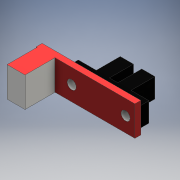
# Autodesk Inventor part: optical endstop
Saved by Autodesk Inventor 2016 SP1 (Build 200210100, 210)
## iProperties
Created: 2016-04-16
Part Number: optical endstop
Material: Generic
Document SubType Name: Modeling
Designer: ubik
Density: 1 g/cm^3
Appearance: Default
Author: ubik
Autodesk Inventor part; units mm, degrees
ref_plane "YZ Plane" through (0, 0, 0) normal (1, 0, 0) x (0, 1, 0)
ref_plane "XZ Plane" through (0, 0, 0) normal (0, 1, 0) x (-1, 0, 0)
ref_plane "XY Plane" through (0, 0, 0) normal (0, 0, 1) x (1, 0, 0)
sketch "Sketch1" plane through (0, 0, 0) normal (0, 0, 1) x (1, 0, 0)
  line L0 (-11.8, 0) -> (-11.8, 3)
  line L1 (-11.8, 3) -> (-5.8, 3)
  line L2 (-5.8, 3) -> (-5.8, 11)
  line L3 (-5.8, 11) -> (-1.4, 11)
  line L4 (-1.4, 11) -> (-1.4, 3)
  line L5 (-1.4, 3) -> (1.4, 3)
  line L6 (1.4, 3) -> (1.4, 11)
  line L7 (1.4, 11) -> (5.8, 11)
  line L8 (5.8, 11) -> (5.8, 3)
  line L9 (5.8, 3) -> (11.8, 3)
  line L10 (11.8, 3) -> (11.8, 0)
  line L11 (11.8, 0) -> (-11.8, 0)
  point P0 (0, 0)
  dimension "d0" = 3
  dimension "d1" = 6
  dimension "d2" = 8
  dimension "d3" = 4.4
  dimension "d4" = 2.8
  dimension "d5" = 4.4
  dimension "d6" = 6
  dimension "d7" = 1.4
  dimension "d8" = 0
  constraints: 24 end point, 8 perpendicular, 6 point on line, 1 vertical
  measures "d0" distance of L0.start L0.end
  measures "d1" distance of L0.end L1.end
  measures "d2" distance of L1.end L2.end
  measures "d3" distance of L2.end L3.end
  measures "d4" distance of L4.end L5.end
  measures "d5" distance of L6.end L7.end
  measures "d6" distance of L8.end L9.end
  measures "d7" distance from line of point (0, 0) L4
  measures "d8" distance from line of point (0, 0) L11
extrude "Extrusion1" add sketch "Sketch1" along normal blind 6.5
sketch "Sketch2" plane through (-11.8, 0, 0) normal (0, -1, 0) x (1, 0, 0)
  circle A0 centre (2.8, 3.25) radius 1.5
  circle A1 centre (20.8, 3.25) radius 1.5
  line L0 (23.6, 0) -> (23.6, 6.5) projected
  line L1 (0, 0) -> (0, 6.5) projected
  line L2 (23.6, 0) -> (0, 0) projected
  line L3 (0, 6.5) -> (23.6, 6.5) projected
  line L4 (11.8, 17.7341) -> (11.8, -9.1991) construction
  line L5 (10.4, 0) -> (10.4, 6.5) construction
  line L6 (13.2, 0) -> (13.2, 6.5) construction
  point P0 (11.8, 0)
  dimension "d11" = 3
  dimension "d12" = 3
  dimension "d13" = 18
  dimension "d14" = 23.6
  dimension "d15" = 2.8
  dimension "d16" = 6.5
  dimension "d17" = 3.25
  dimension "d18" = 3.25
  dimension "d34" = 2.8
  dimension "d35" = 1.4
  constraints: 2 centre point, 2 end point, 1 vertical
  measures "d11" diameter of A0
  measures "d12" diameter of A1
  measures "d13" distance of A1.centre A0.centre
  measures "d14" distance between parallel lines of L0 L1
  measures "d15" distance from line of L1 A0.centre
  measures "d16" distance between parallel lines of L2 L3
  measures "d17" distance from line of L3 A0.centre
  measures "d18" distance from line of A1.centre L3
  measures "d34" distance between parallel lines of L5 L6
  measures "d35" distance between parallel lines of L4 L6
extrude "Extrusion2" cut sketch "Sketch2" against normal through all contours A0 | A1
sketch "Sketch3" plane through (-11.8, 0, 0) normal (0, -1, 0) x (1, 0, 0)
  line L0 (-9.1, 8.25) -> (23.9, 8.25)
  line L1 (23.9, 8.25) -> (23.9, -1.75)
  line L2 (23.9, -1.75) -> (-9.1, -1.75)
  line L3 (-9.1, -1.75) -> (-9.1, 8.25)
  line L4 (23.6, 0) -> (23.6, 6.5) projected
  line L5 (23.6, 0) -> (0, 0) projected
  line L6 (0, 6.5) -> (23.6, 6.5) projected
  circle A0 centre (2.8, 3.25) radius 1.5 projected
  circle A1 centre (20.8, 3.25) radius 1.5 projected
  point P0 (11.8, 0)
  dimension "d21" = 10
  dimension "d22" = 33
  dimension "d23" = 0.3
  dimension "d24" = 6.5
  dimension "d25" = 1.75
  constraints: 8 end point, 2 parallel, 1 horizontal, 1 perpendicular
  measures "d21" distance of L0.end L1.end
  measures "d22" distance of L0.start L0.end
  measures "d23" distance between parallel lines of L4 L1
  measures "d24" distance between parallel lines of L5 L6
  measures "d25" distance between parallel lines of L6 L0
extrude "Extrusion3" add sketch "Sketch3" along normal blind 2
sketch "Sketch4" plane through (-11.8, -2, 0) normal (0, -1, 0) x (1, 0, 0)
  line L0 (-8.8, 8.25) -> (-2.8, 8.25)
  line L1 (-2.8, 8.25) -> (-2.8, -1.75)
  line L2 (-2.8, -1.75) -> (-8.8, -1.75)
  line L3 (-8.8, -1.75) -> (-8.8, 8.25)
  line L4 (-9.1, -1.75) -> (23.9, -1.75) projected
  line L5 (-9.1, -1.75) -> (-9.1, 8.25) projected
  point P0 (11.8, 0)
  dimension "d28" = 10
  dimension "d29" = 6
  dimension "d30" = 0
  dimension "d31" = 0.3
  constraints: 8 end point, 2 parallel, 1 horizontal, 1 perpendicular
  measures "d28" distance of L2.end L0.start
  measures "d29" distance of L0.start L0.end
  measures "d30" distance between parallel lines of L4 L2
  measures "d31" distance between parallel lines of L5 L3
extrude "Extrusion4" add sketch "Sketch4" along normal blind 10
equation "\"d7\" = 0.5 * d4"
equation "\"d15\" = -0.5 * d13 + 0.5 * d14"
equation "\"d17\" = 0.5 * d16"
equation "\"d18\" = d17"
equation "\"d25\" = -0.5 * d24 + 0.5 * d21"
body "Solid1"
